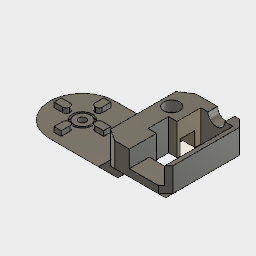
Hip Cross (x4) (Autodesk Fusion 360 design; units mm, degrees)
Autodesk Fusion 360 part; units mm, degrees
note: some values were not read from the file. Set by a fixed rule: which sketch regions a step uses.
sketch "Sketch1" plane through (0, 0, 0) normal (0, 1, 0) x (1, 0, 0)
  circle A0 centre (0, 0) radius 13.5
  line L0 (0.0697, 13.4998) -> (25.0697, 13.4998)
  line L1 (25.0697, 13.4998) -> (25.0697, -13.5002)
  line L2 (25.0697, -13.5002) -> (0.0697, -13.5002)
  line L3 (0.0697, -13.5002) -> (0.0697, 13.4998)
  dimension "d1" = 27
  dimension "d2" = 25
  dimension "d3" = 27
  measures "d1" diameter of A0
  measures "d2" distance of L0.start L0.end
  measures "d3" distance of L0.start L2.end
  measures "d49" distance of L1.end
extrude "Extrude1" add sketch "Sketch1" along normal blind 3 makes body 1
sketch "Sketch2" plane through (0, 3, 0) normal (0, 1, 0) x (-1, 0, 0)
  arc A0 (-0.0697, -13.4998) -> (-0.0697, 13.4998) centre (0, 0) ccw
  line L0 (-0.0697, 13.4998) -> (-0.0697, 13.5002)
  line L1 (-0.0697, 13.5002) -> (-25.0697, 13.5002)
  line L2 (-25.0697, 13.5002) -> (-25.0697, -13.4998)
  line L3 (-25.0697, -13.4998) -> (-0.0697, -13.4998)
  circle A1 centre (0, 0) radius 1.5
  dimension "d7" = 3
  measures "d7" diameter of A1
extrude "Extrude2" cut sketch "Sketch2" against normal blind 10 contours A1 bodies 1
sketch "Sketch3" plane through (0, 3, 0) normal (0, 1, 0) x (-1, 0, 0)
  circle A0 centre (0, 0) radius 1.5
  arc A1 (-0.0697, -13.4998) -> (-0.0697, 13.4998) centre (0, 0) ccw
  line L0 (-0.0697, 13.4998) -> (-0.0697, 13.5002)
  line L1 (-0.0697, 13.5002) -> (-25.0697, 13.5002)
  line L2 (-25.0697, 13.5002) -> (-25.0697, -13.4998)
  line L3 (-25.0697, -13.4998) -> (-0.0697, -13.4998)
  line L4 (0, 0) -> (10.25, 0)
  line L5 (0, 0) -> (-10.25, 0)
  line L6 (10.25, 0) -> (10.25, -1.5) construction
  line L7 (10.25, -1.5) -> (5.25, -1.5)
  line L8 (5.25, -1.5) -> (5.25, 1.5)
  line L9 (5.25, 1.5) -> (10.25, 1.5)
  line L10 (10.25, 1.5) -> (10.25, -1.5)
  line L11 (-10.25, 0) -> (-10.25, -1.5) construction
  line L12 (-10.25, -1.5) -> (-5.25, -1.5)
  line L13 (-5.25, -1.5) -> (-5.25, 1.5)
  line L14 (-5.25, 1.5) -> (-10.25, 1.5)
  line L15 (-10.25, 1.5) -> (-10.25, -1.5)
  line L16 (0, 0) -> (0, -10.25)
  line L17 (0, 0) -> (0, 10.25)
  line L18 (0, 10.25) -> (1.5, 10.25) construction
  line L19 (1.5, 10.25) -> (-1.5, 10.25)
  line L20 (-1.5, 10.25) -> (-1.5, 5.25)
  line L21 (-1.5, 5.25) -> (1.5, 5.25)
  line L22 (1.5, 5.25) -> (1.5, 10.25)
  line L23 (0, -10.25) -> (-1.5, -10.25) construction
  line L24 (-1.5, -10.25) -> (1.5, -10.25)
  line L25 (1.5, -10.25) -> (1.5, -5.25)
  line L26 (1.5, -5.25) -> (-1.5, -5.25)
  line L27 (-1.5, -5.25) -> (-1.5, -10.25)
  dimension "d10" = 10.25
  dimension "d11" = 10.25
  dimension "d12" = 1.5
  dimension "d13" = 3
  dimension "d14" = 5
  dimension "d15" = 1.5
  dimension "d16" = 5
  dimension "d17" = 3
  dimension "d18" = 10.25
  dimension "d19" = 10.25
  dimension "d20" = 1.5
  dimension "d21" = 3
  dimension "d22" = 5
  dimension "d23" = 1.5
  dimension "d24" = 3
  dimension "d25" = 5
  measures "d10" distance of A0.centre L4.end
  measures "d11" distance of A0.centre L5.end
  measures "d12" distance of L4.end L6.end
  measures "d13" distance of L6.end L9.end
  measures "d14" distance of L6.end L7.end
  measures "d15" distance of L5.end L11.end
  measures "d16" distance of L11.end L12.end
  measures "d17" distance of L11.end L14.end
  measures "d18" distance of A0.centre L16.end
  measures "d19" distance of A0.centre L17.end
  measures "d20" distance of L17.end L18.end
  measures "d21" distance of L18.end L19.end
  measures "d22" distance of L18.end L21.end
  measures "d23" distance of L16.end L23.end
  measures "d24" distance of L23.end L24.end
  measures "d25" distance of L23.end L26.end
extrude "Extrude3" add sketch "Sketch3" along normal blind 2 contours L4 L8 L9 L10 | L4 L7 L8 L10 | L5 L12 L13 L15 | L5 L13 L14 L15 | L16 L24 L25 L26 | L16 L24 L26 L27 | L17 L19 L20 L21 | L17 L19 L21 L22 bodies 1
fillet "Fillet1" radius 1.35 1 edges at (-5.25, 4, 1.5) on bodies 1
fillet "Fillet2" radius 1.35 7 edges at (-5.25, 4, -1.5) (-1.5, 4, -5.25) (1.5, 4, -5.25) (5.25, 4, -1.5) (5.25, 4, 1.5) (1.5, 4, 5.25) (-1.5, 4, 5.25) on bodies 1
sketch "Sketch4" plane through (0, 3, 0) normal (0, 1, 0) x (-1, 0, 0)
  line L0 (0.15, 5.25) -> (-0.15, 5.25)
  arc A0 (-1.5, 6.6) -> (-0.15, 5.25) centre (-0.15, 6.6) ccw
  line L1 (-1.5, 6.6) -> (-1.5, 10.25)
  line L2 (-1.5, 10.25) -> (1.5, 10.25)
  line L3 (1.5, 10.25) -> (1.5, 6.6)
  arc A1 (0.15, 5.25) -> (1.5, 6.6) centre (0.15, 6.6) ccw
  line L4 (10.25, 1.5) -> (10.25, -1.5)
  line L5 (10.25, -1.5) -> (6.6, -1.5)
  arc A2 (5.25, -0.15) -> (6.6, -1.5) centre (6.6, -0.15) ccw
  line L6 (5.25, -0.15) -> (5.25, 0.15)
  arc A3 (6.6, 1.5) -> (5.25, 0.15) centre (6.6, 0.15) ccw
  line L7 (6.6, 1.5) -> (10.25, 1.5)
  line L8 (-0.15, -5.25) -> (0.15, -5.25)
  arc A4 (1.5, -6.6) -> (0.15, -5.25) centre (0.15, -6.6) ccw
  line L9 (1.5, -6.6) -> (1.5, -10.25)
  line L10 (1.5, -10.25) -> (-1.5, -10.25)
  line L11 (-1.5, -10.25) -> (-1.5, -6.6)
  arc A5 (-0.15, -5.25) -> (-1.5, -6.6) centre (-0.15, -6.6) ccw
  line L12 (-10.25, 1.5) -> (-6.6, 1.5)
  arc A6 (-5.25, 0.15) -> (-6.6, 1.5) centre (-6.6, 0.15) ccw
  line L13 (-5.25, 0.15) -> (-5.25, -0.15)
  arc A7 (-6.6, -1.5) -> (-5.25, -0.15) centre (-6.6, -0.15) ccw
  line L14 (-6.6, -1.5) -> (-10.25, -1.5)
  line L15 (-10.25, -1.5) -> (-10.25, 1.5)
  circle A8 centre (0, 0) radius 1.5
  arc A9 (-0.0697, -13.4998) -> (-0.0697, 13.4998) centre (0, 0) ccw
  line L16 (-0.0697, 13.4998) -> (-0.0697, 13.5002)
  line L17 (-0.0697, 13.5002) -> (-25.0697, 13.5002)
  line L18 (-25.0697, 13.5002) -> (-25.0697, -13.4998)
  line L19 (-25.0697, -13.4998) -> (-0.0697, -13.4998)
  circle A10 centre (0, 0) radius 3.4
  circle A11 centre (0, 0) radius 4.125
  dimension "d31" = 6.8
  dimension "d32" = 8.25
  measures "d31" diameter of A10
  measures "d32" diameter of A11
extrude "Extrude4" cut sketch "Sketch4" against normal blind 1 contours A11 bodies 1
sketch "Sketch5" plane through (0, 3, 0) normal (0, 1, 0) x (-1, 0, 0)
  arc A0 (-0.0697, -13.4998) -> (-0.0697, 13.4998) centre (0, 0) ccw
  line L0 (-0.0697, 13.4998) -> (-0.0697, 13.5002)
  line L1 (-0.0697, 13.5002) -> (-25.0697, 13.5002)
  line L2 (-25.0697, 13.5002) -> (-25.0697, -13.4998)
  line L3 (-25.0697, -13.4998) -> (-0.0697, -13.4998)
  line L4 (-10.25, 1.5) -> (-6.6, 1.5)
  arc A1 (-5.25, 0.15) -> (-6.6, 1.5) centre (-6.6, 0.15) ccw
  line L5 (-5.25, 0.15) -> (-5.25, -0.15)
  arc A2 (-6.6, -1.5) -> (-5.25, -0.15) centre (-6.6, -0.15) ccw
  line L6 (-6.6, -1.5) -> (-10.25, -1.5)
  line L7 (-10.25, -1.5) -> (-10.25, 1.5)
  line L8 (-0.15, -5.25) -> (0.15, -5.25)
  arc A3 (1.5, -6.6) -> (0.15, -5.25) centre (0.15, -6.6) ccw
  line L9 (1.5, -6.6) -> (1.5, -10.25)
  line L10 (1.5, -10.25) -> (-1.5, -10.25)
  line L11 (-1.5, -10.25) -> (-1.5, -6.6)
  arc A4 (-0.15, -5.25) -> (-1.5, -6.6) centre (-0.15, -6.6) ccw
  line L12 (10.25, 1.5) -> (10.25, -1.5)
  line L13 (10.25, -1.5) -> (6.6, -1.5)
  arc A5 (5.25, -0.15) -> (6.6, -1.5) centre (6.6, -0.15) ccw
  line L14 (5.25, -0.15) -> (5.25, 0.15)
  arc A6 (6.6, 1.5) -> (5.25, 0.15) centre (6.6, 0.15) ccw
  line L15 (6.6, 1.5) -> (10.25, 1.5)
  line L16 (0.15, 5.25) -> (-0.15, 5.25)
  arc A7 (-1.5, 6.6) -> (-0.15, 5.25) centre (-0.15, 6.6) ccw
  line L17 (-1.5, 6.6) -> (-1.5, 10.25)
  line L18 (-1.5, 10.25) -> (1.5, 10.25)
  line L19 (1.5, 10.25) -> (1.5, 6.6)
  arc A8 (0.15, 5.25) -> (1.5, 6.6) centre (0.15, 6.6) ccw
  circle A9 centre (0, 0) radius 4.125
  line L20 (-25.0697, 0.0002) -> (-25.0697, -16.7498) construction
  line L21 (-25.0697, -16.7498) -> (-51.0697, -16.7498)
  line L22 (-51.0697, -16.7498) -> (-51.0697, 16.7502)
  line L23 (-51.0697, 16.7502) -> (-25.0697, 16.7502)
  line L24 (-25.0697, 16.7502) -> (-25.0697, -16.7498)
  dimension "d35" = 16.75
  dimension "d36" = 26
  dimension "d37" = 33.5
  measures "d35" distance of L20.start L20.end
  measures "d36" distance of L20.end L21.end
  measures "d37" distance of L20.end L23.end
extrude "Extrude5" add sketch "Sketch5" along normal blind 13 separate body contours L2 L21 L22 L23 L24 makes body 2
move_body "MoveBody1" bodies 2 to x (1, 0, 0) y (0, 1, 0) z (0, 0, 1) at (0, 3, 0)
sketch "Sketch6" plane through (0, 0, 13.5002) normal (0, 0, 1) x (1, 0, 0)
  line L0 (0.0697, 0) -> (25.0697, 0)
  line L1 (25.0697, 0) -> (25.0697, 3)
  line L2 (25.0697, 3) -> (0.0697, 3)
  line L3 (0.0697, 3) -> (0.0697, 0)
  line L4 (25.0697, 0) -> (31.0697, 6)
  line L5 (25.0697, 0) -> (36.3342, 0) construction
  line L6 (25.0697, 6) -> (31.0697, 6)
  line L7 (25.0697, 0) -> (25.0697, 6)
  point P0 (25.0697, 6)
  dimension "d40" = 45
  measures "d40" angle of L4 L5
extrude "Extrude6" add sketch "Sketch6" against normal blind 27 contours L1 L4 L6 L7 bodies 1 2
sketch "Sketch7" plane through (0, 19, 0) normal (0, 1, 0) x (-1, 0, 0)
  line L0 (-25.0697, 16.7502) -> (-51.0697, 16.7502)
  line L1 (-51.0697, 16.7502) -> (-51.0697, -16.7498)
  line L2 (-51.0697, -16.7498) -> (-25.0697, -16.7498)
  line L3 (-25.0697, -16.7498) -> (-25.0697, 16.7502)
  line L4 (-25.0697, 16.7502) -> (-36.0697, 16.7502) construction
  line L5 (-36.0697, 16.7502) -> (-49.3197, 16.7502)
  line L6 (-49.3197, 16.7502) -> (-49.3197, -12.7498)
  line L7 (-49.3197, -12.7498) -> (-36.0697, -12.7498)
  line L8 (-36.0697, -12.7498) -> (-36.0697, 16.7502)
  dimension "d44" = 11
  dimension "d45" = 29.5
  dimension "d46" = 13.25
  measures "d44" distance of L0.start L4.end
  measures "d45" distance of L4.end L7.end
  measures "d46" distance of L4.end L5.end
extrude "Extrude7" cut sketch "Sketch7" against normal blind 7 contours L0 L5 L6 L7 L8 bodies 1
sketch "Sketch8" plane through (0, 19, 0) normal (0, 1, 0) x (-1, 0, 0)
  line L0 (-36.0697, 16.7502) -> (-36.0697, -12.7498)
  line L1 (-36.0697, -12.7498) -> (-49.3197, -12.7498)
  line L2 (-49.3197, -12.7498) -> (-49.3197, 16.7502)
  line L3 (-49.3197, 16.7502) -> (-51.0697, 16.7502)
  line L4 (-51.0697, 16.7502) -> (-51.0697, -16.7498)
  line L5 (-51.0697, -16.7498) -> (-25.0697, -16.7498)
  line L6 (-25.0697, -16.7498) -> (-25.0697, 16.7502)
  line L7 (-25.0697, 16.7502) -> (-36.0697, 16.7502)
  line L8 (-25.0697, -16.7498) -> (-29.5697, -16.7498) construction
  line L9 (-29.5697, -16.7498) -> (-29.576, -7.2498) construction
  circle A0 centre (-29.576, -7.2498) radius 3.25
  dimension "d49" = 4.5
  dimension "d50" = 9.5
  dimension "d51" = 6.5
  measures "d49" distance of L5.end L8.end
  measures "d50" distance of L8.end L9.end
  measures "d51" diameter of A0
extrude "Extrude8" cut sketch "Sketch8" against normal blind 4.4 contours A0 bodies 1
sketch "Sketch9" plane through (0, 14.6, 0) normal (0, 1, 0) x (-1, 0, 0)
  circle A0 centre (-29.576, -7.2498) radius 3.25
  circle A1 centre (-29.576, -7.2498) radius 1.75
  dimension "d57" = 3.5
  measures "d57" diameter of A1
extrude "Extrude9" cut sketch "Sketch9" against normal blind 15 contours A1 bodies 1
sketch "Sketch10" plane through (0, 19, 0) normal (0, 1, 0) x (-1, 0, 0)
  circle A0 centre (-29.576, -7.2498) radius 3.25
  line L0 (-36.0697, 16.7502) -> (-36.0697, -12.7498)
  line L1 (-36.0697, -12.7498) -> (-49.3197, -12.7498)
  line L2 (-49.3197, -12.7498) -> (-49.3197, 16.7502)
  line L3 (-49.3197, 16.7502) -> (-51.0697, 16.7502)
  line L4 (-51.0697, 16.7502) -> (-51.0697, -16.7498)
  line L5 (-51.0697, -16.7498) -> (-25.0697, -16.7498)
  line L6 (-25.0697, -16.7498) -> (-25.0697, 16.7502)
  line L7 (-25.0697, 16.7502) -> (-36.0697, 16.7502)
  line L8 (-36.0697, 1.3059) -> (-32.5697, 1.3059) construction
  line L9 (-32.5697, 1.3059) -> (-32.5697, -2.9441) construction
  line L10 (-32.5697, -2.9441) -> (-36.0697, -2.9441)
  line L11 (-36.0697, -2.9441) -> (-36.0697, 5.5559)
  line L12 (-36.0697, 5.5559) -> (-32.5697, 5.5559)
  line L13 (-32.5697, 5.5559) -> (-32.5697, -2.9441)
  dimension "d62" = 3.5
  dimension "d63" = 4.25
  dimension "d64" = 3.5
  dimension "d65" = 8.5
  measures "d62" distance of L8.start L8.end
  measures "d63" distance of L8.end L9.end
  measures "d64" distance of L9.end L10.end
  measures "d65" distance of L9.end L12.end
extrude "Extrude10" cut sketch "Sketch10" against normal blind 22 contours L0 L10 L11 L12 L13 bodies 1
sketch "Sketch11" plane through (0, 12, 0) normal (0, 1, 0) x (-1, 0, 0)
  line L0 (-36.0697, 5.5559) -> (-36.0697, 16.7502)
  line L1 (-36.0697, 16.7502) -> (-49.3197, 16.7502)
  line L2 (-49.3197, 16.7502) -> (-49.3197, -12.7498)
  line L3 (-49.3197, -12.7498) -> (-36.0697, -12.7498)
  line L4 (-36.0697, -12.7498) -> (-36.0697, -2.9441)
  line L5 (-36.0697, -2.9441) -> (-36.0697, 5.5559)
  line L6 (-49.3197, 16.7502) -> (-49.3197, 8.5002) construction
  line L7 (-49.3197, 8.5002) -> (-36.0697, 8.5002)
  line L8 (-36.0697, 8.5002) -> (-36.0697, 0.0002)
  line L9 (-36.0697, 0.0002) -> (-49.3197, 0.0002)
  line L10 (-49.3197, 0.0002) -> (-49.3197, 8.5002)
  dimension "d68" = 8.25
  dimension "d69" = 13.25
  dimension "d70" = 8.5
  measures "d68" distance of L1.end L6.end
  measures "d69" distance of L6.end L7.end
  measures "d70" distance of L6.end L9.end
extrude "Extrude11" cut sketch "Sketch11" against normal blind 13 contours L0 L2 L5 L7 L8 L9 L10 bodies 1
sketch "Sketch12" plane through (0, 12, 0) normal (0, 1, 0) x (-1, 0, 0)
  line L0 (-36.0697, 0.0002) -> (-49.3197, 0.0002)
  line L1 (-49.3197, 0.0002) -> (-49.3197, -12.7498)
  line L2 (-49.3197, -12.7498) -> (-36.0697, -12.7498)
  line L3 (-36.0697, -12.7498) -> (-36.0697, -2.9441)
  line L4 (-36.0697, -2.9441) -> (-36.0697, 0.0002)
  line L5 (-49.3197, 0.0002) -> (-46.8197, 0.0002) construction
  line L6 (-46.8197, 0.0002) -> (-36.0697, 0.0002)
  line L7 (-36.0697, 0.0002) -> (-36.0697, -12.7498)
  line L8 (-36.0697, -12.7498) -> (-46.8197, -12.7498)
  line L9 (-46.8197, -12.7498) -> (-46.8197, 0.0002)
  dimension "d73" = 2.5
  measures "d73" distance of L0.end L5.end
extrude "Extrude12" cut sketch "Sketch12" against normal blind 16 contours L0 L2 L3 L4 L6 L7 L8 L9 bodies 1
sketch "Sketch13" plane through (0, 0, -16.7498) normal (0, 0, -1) x (-1, 0, 0)
  line L0 (-51.0697, 6) -> (-25.0697, 6)
  line L1 (-25.0697, 6) -> (-25.0697, 19)
  line L2 (-25.0697, 19) -> (-51.0697, 19)
  line L3 (-51.0697, 19) -> (-51.0697, 6)
  line L4 (-51.0697, 19) -> (-42.5197, 19)
  circle A0 centre (-42.5197, 19) radius 3.5
  dimension "d76" = 8.55
  dimension "d77" = 7
  measures "d76" distance of L2.end L4.end
  measures "d77" diameter of A0
extrude "Extrude13" cut sketch "Sketch13" against normal blind 7 contours L2 L4 A0 picked at (-44.84, 18.8261) bodies 1
sketch "Sketch14" plane through (36.0697, 0, 0) normal (1, 0, 0) x (0, 0, -1)
  line L0 (2.9441, 19) -> (2.9441, 6)
  line L1 (2.9441, 6) -> (12.7498, 6)
  line L2 (12.7498, 6) -> (12.7498, 19)
  line L3 (12.7498, 19) -> (2.9441, 19)
sketch "Sketch15" plane through (0, 6, 0) normal (0, -1, 0) x (1, 0, 0)
  line L0 (25.0697, 13.5002) -> (31.0697, 13.5002)
  line L1 (31.0697, -8.1616) -> (31.0697, -13.4998)
  line L2 (31.0697, -13.4998) -> (25.0697, -13.4998)
  line L3 (25.0697, -13.4998) -> (25.0697, -16.7498)
  line L4 (25.0697, -16.7498) -> (51.0697, -16.7498)
  line L5 (51.0697, -16.7498) -> (51.0697, 16.7502)
  line L6 (51.0697, 16.7502) -> (25.0697, 16.7502)
  line L7 (25.0697, 16.7502) -> (25.0697, 13.5002)
  line L8 (46.8197, 0.0002) -> (46.8197, -12.7498)
  line L9 (46.8197, -12.7498) -> (36.0697, -12.7498)
  line L10 (36.0697, -12.7498) -> (36.0697, -2.9441)
  line L11 (36.0697, -2.9441) -> (32.5697, -2.9441)
  line L12 (32.5697, -2.9441) -> (32.5697, 5.5559)
  line L13 (32.5697, 5.5559) -> (36.0697, 5.5559)
  line L14 (36.0697, 5.5559) -> (36.0697, 8.5002)
  line L15 (36.0697, 8.5002) -> (49.3197, 8.5002)
  line L16 (49.3197, 8.5002) -> (49.3197, 0.0002)
  line L17 (49.3197, 0.0002) -> (46.8197, 0.0002)
  line L18 (36.0697, -12.7498) -> (36.0697, -10.2498) construction
  line L19 (36.0697, -10.2498) -> (26.0697, -10.2498)
  line L20 (26.0697, -10.2498) -> (26.0697, -4.2498)
  line L21 (26.0697, -4.2498) -> (36.0697, -4.2498)
  line L22 (36.0697, -4.2498) -> (36.0697, -10.2498)
  arc A0 (31.0697, -8.1616) -> (31.0697, -6.338) centre (29.576, -7.2498) ccw
  line L23 (31.0697, 13.5002) -> (31.0697, -6.338)
  dimension "d82" = 2.5
  dimension "d83" = 6
  measures "d82" distance of L9.end L18.end
  measures "d83" distance of L18.end L21.end
extrude "Extrude14" cut sketch "Sketch15" against normal blind 6.1 contours L1 L19 L20 L21 A0 L23 | L1 L10 L19 L21 L22 A0 L23 bodies 1
extrude "Extrude15" cut 1 faces at (34.4884, 12.1, -7.2498) along direction (0, -1, 0) blind 20 on bodies 1 bodies 1
sketch "Sketch16" plane through (0, 19, 0) normal (0, 1, 0) x (-1, 0, 0)
  line L0 (-39.0197, -12.7498) -> (-39.0197, -16.7498)
  line L1 (-39.0197, -16.7498) -> (-25.0697, -16.7498)
  line L2 (-25.0697, -16.7498) -> (-25.0697, 16.7502)
  line L3 (-25.0697, 16.7502) -> (-36.0697, 16.7502)
  line L4 (-36.0697, 16.7502) -> (-36.0697, 5.5559)
  line L5 (-36.0697, 5.5559) -> (-32.5697, 5.5559)
  line L6 (-32.5697, 5.5559) -> (-32.5697, -2.9441)
  line L7 (-32.5697, -2.9441) -> (-36.0697, -2.9441)
  line L8 (-36.0697, -2.9441) -> (-36.0697, -12.7498)
  line L9 (-36.0697, -12.7498) -> (-39.0197, -12.7498)
  circle A0 centre (-29.576, -7.2498) radius 3.25
  line L10 (-25.0697, 16.7502) -> (-30.0697, 16.7502)
  line L11 (-25.0697, 13.5002) -> (-30.0697, 16.7502)
  line L12 (-25.0697, -16.7498) -> (-30.0697, -16.7498)
  line L13 (-30.0697, -16.7498) -> (-25.0697, -13.4998)
  point P0 (-25.0697, 13.5002)
  point P1 (-25.0697, -13.4998)
  dimension "d88" = 5
  dimension "d89" = 5
  measures "d88" distance of L2.end L10.end
  measures "d89" distance of L1.end L12.end
extrude "Extrude16" cut sketch "Sketch16" against normal blind 25 contours L1 L2 L12 L13 | L2 L3 L10 L11 bodies 1
sketch "Sketch17" plane through (0, 6, 0) normal (0, -1, 0) x (1, 0, 0)
  line L0 (30.0697, 16.7502) -> (25.0697, 13.5002)
  line L1 (25.0697, 13.5002) -> (31.0697, 13.5002)
  line L2 (31.0697, 13.5002) -> (31.0697, -4.2498)
  line L3 (31.0697, -4.2498) -> (36.0697, -4.2498)
  line L4 (36.0697, -4.2498) -> (36.0697, -2.9441)
  line L5 (36.0697, -2.9441) -> (32.5697, -2.9441)
  line L6 (32.5697, -2.9441) -> (32.5697, 5.5559)
  line L7 (32.5697, 5.5559) -> (36.0697, 5.5559)
  line L8 (36.0697, 5.5559) -> (36.0697, 8.5002)
  line L9 (36.0697, 8.5002) -> (49.3197, 8.5002)
  line L10 (49.3197, 8.5002) -> (49.3197, 0.0002)
  line L11 (49.3197, 0.0002) -> (46.8197, 0.0002)
  line L12 (46.8197, 0.0002) -> (46.8197, -12.7498)
  line L13 (46.8197, -12.7498) -> (36.0697, -12.7498)
  line L14 (36.0697, -12.7498) -> (36.0697, -10.2498)
  line L15 (36.0697, -10.2498) -> (31.0697, -10.2498)
  line L16 (31.0697, -10.2498) -> (31.0697, -13.4998)
  line L17 (31.0697, -13.4998) -> (25.0697, -13.4998)
  line L18 (25.0697, -13.4998) -> (30.0697, -16.7498)
  line L19 (30.0697, -16.7498) -> (51.0697, -16.7498)
  line L20 (51.0697, -16.7498) -> (51.0697, 16.7502)
  line L21 (51.0697, 16.7502) -> (30.0697, 16.7502)
  line L22 (25.0697, 13.5002) -> (30.0697, 16.7502)
  line L23 (30.0697, 13.5002) -> (25.0697, 13.5002)
  line L24 (30.0697, 13.5002) -> (30.0697, 16.7502)
  line L25 (25.0697, -13.4998) -> (30.0697, -13.4998)
  line L26 (30.0697, -13.4998) -> (30.0697, -16.7498)
  line L27 (30.0697, -16.7498) -> (25.0697, -13.4998)
  dimension "d92" = 5
  measures "d92" distance of L17.end L25.end
chamfer "Chamfer1" distance 3 angle 45 3 edges at (12.5697, 0, 13.5002) (12.5697, 0, -13.4998) (-13.5, 0, 0) on bodies 1
chamfer "Chamfer5" distance 5 angle 45 1 edges at (25.0697, 3, 0.0002) on bodies 1
chamfer "Chamfer6" distance 3 angle 45 5 edges at (40.5697, 6, 16.7502) (51.0697, 12.5, 16.7502) (51.0697, 6, 0.0002) (40.5697, 6, -16.7498) (51.0697, 12.5, -16.7498) on bodies 1
equation "d2 = PCBSeparation"
equation "d4 = BottomThickness"
equation "BottomThickness = 3 mm"
equation "d28 = CrossFit"
equation "CrossFit = 1.35 mm"
equation "d30 = CrossFit"
equation "PCBSeparation = 25 mm"
equation "d49 = HolePosX"
equation "d50 = HolePosY"
equation "d51 = HoleSize"
equation "HolePosX = 4.5 mm"
equation "HolePosY = 9.5 mm"
equation "HoleSize = 6.5 mm"
equation "d55 = -SpacerHoleDepth"
equation "d57 = ScrewHoleSize"
equation "ScrewHoleSize = 3.5 mm"
equation "d103 = Chamfer3"
equation "Chamfer3 = 3 mm"
equation "ChamferStrength = 5 mm"
equation "d109 = ChamferStrength"
equation "d110 = Chamfer3"
equation "SpacerHoleDepth = 4.4 mm"
